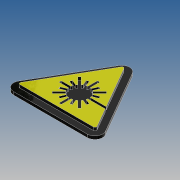
# Autodesk Inventor part: P129
Saved by Autodesk Inventor 2019 (Build 230136000, 136)
## iProperties
Created: 2017-01-31
Part Number: P129
Material: Generic
Document SubType Name: Modeling
Designer: serge.amoos
Density: 1 g/cm^3
Appearance: Smooth - Black
Description: Signal laser
Author: serge.amoos
Autodesk Inventor part; units mm, degrees
ref_plane "YZ Plane" through (0, 0, 0) normal (1, 0, 0) x (0, 1, 0)
ref_plane "XZ Plane" through (0, 0, 0) normal (0, 1, 0) x (-1, 0, 0)
ref_plane "XY Plane" through (0, 0, 0) normal (0, 0, 1) x (1, 0, 0)
sketch "Sketch1" plane through (0, 0, 0) normal (0, 0, 1) x (1, 0, 0)
  line L0 (-9.1, 0) -> (9.1, 0) construction
  line L1 (0, -6.0044) -> (0, 9.7572) construction
  line L2 (0, 7.5056) -> (6.5, -3.7528)
  line L3 (6.5, -3.7528) -> (-6.5, -3.7528)
  line L4 (-6.5, -3.7528) -> (0, 7.5056)
  point P0 (0, 0)
  point P1 (0, 0)
  dimension "d0" = 13
  constraints: 6 end point, 1 coincident, 1 point on line, 7 other
  measures "d0" distance of L2.end L3.end
extrude "Extrusion1" add sketch "Sketch1" along normal blind 0.4
fillet "Fillet1" radius 1 3 edges at (-6.5, -3.7528, 0.2) (6.5, -3.7528, 0.2) (0, 7.5056, 0.2)
sketch "Sketch2" plane through (0, 0, 0.4) normal (0, 0, 1) x (1, 0, 0)
  arc A0 (-5.634, -2.2528) -> (-4.7679, -3.7528) centre (-4.7679, -2.7528) ccw projected
  line L0 (-5.634, -2.2528) -> (-0.866, 6.0056) projected
  arc A1 (0.866, 6.0056) -> (-0.866, 6.0056) centre (0, 5.5056) ccw projected
  line L1 (0.866, 6.0056) -> (5.634, -2.2528) projected
  arc A2 (4.7679, -3.7528) -> (5.634, -2.2528) centre (4.7679, -2.7528) ccw projected
  line L2 (4.7679, -3.7528) -> (-4.7679, -3.7528) projected
  line L3 (-0.1732, 5.6056) -> (-4.9412, -2.6528)
  arc A3 (-4.9412, -2.6528) -> (-4.7679, -2.9528) centre (-4.7679, -2.7528) ccw
  line L4 (-4.7679, -2.9528) -> (4.7679, -2.9528)
  arc A4 (4.7679, -2.9528) -> (4.9412, -2.6528) centre (4.7679, -2.7528) ccw
  line L5 (4.9412, -2.6528) -> (0.1732, 5.6056)
  arc A5 (0.1732, 5.6056) -> (-0.1732, 5.6056) centre (0, 5.5056) ccw
  circle A6 centre (0, 0) radius 1.25
  dimension "d4" = 0.8
  dimension "d5" = 2.5
  constraints: 6 end point, 6 point on circle, 4 centre point, 1 coincident, 5 other
  measures "d4" distance between parallel lines of L3 L0
  measures "d5" diameter of A6
extrude "Extrusion2" add sketch "Sketch2" along normal blind 0.4 contours A5 L5 A4 L4 A3 L3
sketch "Sketch3" plane through (0, 0, 0.8) normal (0, 0, 1) x (1, 0, 0)
  line L0 (-8.0751, 0) -> (8.0751, 0) construction
  line L1 (0, -5.8044) -> (0, 8.5572) construction
  circle A0 centre (0, 0) radius 1.25 construction
  line L2 (-0.15, 2.5) -> (0.15, 2.5)
  line L3 (0.15, 2.5) -> (0.15, -0.4687)
  line L4 (0.15, -0.4687) -> (-0.15, -0.4687)
  line L5 (-0.15, -0.4687) -> (-0.15, 2.5)
  point P0 (0, 2.5)
  dimension "d8" = 0.3
  dimension "d9" = 2.5
  constraints: 8 end point, 2 parallel, 1 horizontal, 1 midpoint, 1 perpendicular, 1 point on line
  measures "d8" distance of L2.start L2.end
  measures "d9" distance between parallel lines of L0 L2
extrude "Extrusion3" cut sketch "Sketch3" against normal blind 0.4
pattern_circular "Circular Pattern1" count 8 over 360 about axis through (0, 0, -10) along (0, 0, 1) of "Extrusion3"
sketch "Sketch4" plane through (0, 0, 0.8) normal (0, 0, 1) x (1, 0, 0)
  line L0 (0, -5.8044) -> (0, 8.5572) construction
  line L1 (-8.0751, 0) -> (8.0751, 0) construction
  line L2 (0, 0) -> (1.8051, 4.3579) construction
  line L3 (0.6268, 1.9052) -> (0.9039, 1.7904)
  line L4 (0.9039, 1.7904) -> (0.2506, 0.2129)
  line L5 (0.2506, 0.2129) -> (-0.0266, 0.3277)
  line L6 (-0.0266, 0.3277) -> (0.6268, 1.9052)
  point P0 (0.7654, 1.8478)
  dimension "d15" = 22.5
  dimension "d16" = 0.3
  dimension "d17" = 2
  constraints: 10 end point, 2 parallel, 2 perpendicular, 1 midpoint, 1 point on line
  measures "d15" angle of L0 L2
  measures "d16" distance of L3.start L3.end
  measures "d17" distance from line of L3 L2.start
extrude "Extrusion4" cut sketch "Sketch4" against normal blind 0.4
pattern_circular "Circular Pattern2" count 8 over 360 about axis through (0, 0, -10) along (0, 0, 1) of "Extrusion4"
sketch "Sketch5" plane through (0, 0, 0.8) normal (0, 0, 1) x (1, 0, 0)
  line L0 (1.241, 0.15) -> (2.5, 0.15) construction
  line L1 (2.5, -0.15) -> (1.241, -0.15) construction
  line L2 (2.5, 0.15) -> (5.6384, 0.15)
  line L3 (5.6384, 0.15) -> (5.6384, -0.15)
  line L4 (5.6384, -0.15) -> (2.5, -0.15)
  line L5 (2.5, -0.15) -> (2.5, 0.15)
  point P0 (0, 0)
  constraints: 8 end point, 2 parallel, 1 collinear, 1 horizontal, 1 perpendicular
extrude "Extrusion5" cut sketch "Sketch5" against normal blind 0.4
body "Solid1"
